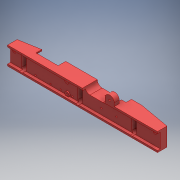
# Autodesk Inventor part: xtion_custom
Saved by Autodesk Inventor 2017 (Build 210142000, 142)
## iProperties
Created: 2016-11-20
Part Number: xtion_custom
Material: PC/ABS Plastic
Document SubType Name: Modeling
Designer: Alistair
Density: 0.357273 g/cm^3
Appearance: Smooth - Red
Author: Alistair
## iProperties of the stored document xtion_custom_3DPrint.ipt
Created: 2016-11-26
Part Number: xtion_custom_3DPrint
Material: Generic
Document SubType Name: Modeling
Designer: Alistair
Density: 1 g/cm^3
Appearance: Default
Author: Alistair
Autodesk Inventor part; units mm, degrees
ref_plane "YZ Plane" through (0, 0, 0) normal (1, 0, 0) x (0, 1, 0)
ref_plane "XZ Plane" through (0, 0, 0) normal (0, 1, 0) x (-1, 0, 0)
sketch "Sketch1" plane through (0, 0, 0) normal (0, 0, 1) x (1, 0, 0)
  line L0 (-10.5, 14) -> (-30.5, 14) projected
  line L1 (-30.5, 5.7) -> (-59, 5.7) construction
  line L2 (36.089, 8.08) -> (32.189, 8.08) projected
  line L3 (19.389, 8.08) -> (15.889, 8.08) projected
  line L4 (-10.5, 14) -> (14.0458, 14)
  line L5 (14.0458, 14) -> (14.0458, 8.08)
  line L6 (14.0458, 8.08) -> (15.889, 8.08)
  line L7 (19.389, 8.08) -> (19.389, 3.1279)
  line L8 (19.389, 3.1279) -> (32.189, 3.1279)
  line L9 (32.189, 3.1279) -> (32.189, 8.08)
  line L10 (36.089, 8.08) -> (37.2137, 8.08)
  line L11 (37.2137, 8.08) -> (37.2137, 14)
  line L12 (37.2137, 14) -> (48.426, 14)
  line L13 (48.426, 14) -> (82, 8.08)
  line L14 (82, 8.08) -> (82, -2.3)
  line L15 (82, -2.3) -> (-82, -2.3)
  line L16 (-82, -2.3) -> (-82, 8.08)
  line L17 (82, 0) -> (82, 29) projected
  line L18 (-82, 0) -> (-82, 29) projected
  line L19 (-82, 8.08) -> (-59, 12.1355)
  line L20 (-59, 5.7) -> (-59, 12.1355)
  line L21 (-34.7264, 5.7) -> (-34.7264, 14)
  line L22 (-34.7264, 14) -> (-30.5, 14)
  line L23 (-34.7264, 5.7) -> (-59, 5.7)
  line L24 (82, 8.08) -> (-65.0862, 8.08) construction
  point P0 (0, 0)
  dimension "d0" = 100
  dimension "d1" = 0
  dimension "d2" = 0
  dimension "d3" = 100
  dimension "d6" = 8
  constraints: 38 end point, 7 perpendicular, 6 point on line, 3 vertical, 2 collinear, 2 horizontal, 1 parallel
  measures "d0" angle of L13 L14
  measures "d1" distance between parallel lines of L14 L17
  measures "d2" distance between parallel lines of L16 L18
  measures "d3" angle of L19 L16
  measures "d6" distance between parallel lines of L15 L1
extrude "Extrusion1" add sketch "Sketch1" along normal mid plane 20
sketch "Sketch2" plane through (-82, -2.3, 10) normal (0, -1, 0) x (1, 0, 0)
  line L0 (164, -20) -> (164, 0) projected
  line L1 (0, 0) -> (164, 0) projected
  line L2 (0, -20) -> (0, 0) projected
  line L3 (164, -20) -> (0, -20) projected
  line L4 (0, -20) -> (0, 0) projected
  line L5 (0, -2) -> (164, -2)
  line L6 (164, -2) -> (164, -18)
  line L7 (164, -18) -> (0, -18)
  line L8 (0, -18) -> (0, -2)
  line L9 (82, -10) -> (90.9812, -10) construction
  point P0 (164, -10)
  dimension "d7" = 16
  constraints: 10 end point, 3 point on line, 2 horizontal, 2 parallel, 1 midpoint, 1 perpendicular
  measures "d7" distance between parallel lines of L5 L7
extrude "Extrusion2" cut sketch "Sketch2" against normal blind 3 contours L7 L2 L5 L0
sketch "Sketch3" plane through (-82, 0.7, 10) normal (0, -1, 0) x (1, 0, 0)
  circle A0 centre (5.4792, -3.8) radius 2
  line L0 (5.4792, -3.8) -> (159.4792, -3.8) construction
  circle A1 centre (159.4792, -3.8) radius 2
  line L1 (164, -2) -> (164, -18) projected
  line L2 (0, -2) -> (164, -2) projected
  line L3 (0, -18) -> (0, -2) projected
  line L4 (164, -18) -> (0, -18) projected
  point P0 (82, -10)
  dimension "d10" = 4
  dimension "d11" = 154
  dimension "d12" = 4
  dimension "d13" = 1.8
  constraints: 2 centre point, 2 end point, 1 coincident, 1 horizontal
  measures "d10" diameter of A0
  measures "d11" distance of L0.start L0.end
  measures "d12" diameter of A1
  measures "d13" distance between parallel lines of L0 L2
extrude "Extrusion3" add sketch "Sketch3" along normal blind 1.2 contours A0 L2 | L2 A0 | L2 A1 | A1 L2
sketch "Sketch4" plane through (-34.7264, 14, 10) normal (0, 1, 0) x (1, 0, 0)
  line L0 (0, 20) -> (0, 0) projected
  line L1 (48.7722, 0) -> (0, 0) projected
  line L2 (48.7722, 20) -> (48.7722, 0) projected
  line L3 (0, 20) -> (48.7722, 20) projected
  line L4 (27.8056, 3.9) -> (27.8056, 16.1) projected
  line L5 (30.6056, 16.1) -> (30.6056, 3.9) projected
  line L6 (29.2376, 3.9) -> (29.2376, 16.1) construction
  line L7 (31.7376, 3.9) -> (31.7376, 16.1)
  line L8 (26.7376, 16.1) -> (26.7376, 3.9)
  arc A0 (26.7376, 3.9) -> (31.7376, 3.9) centre (29.2376, 3.9) ccw
  arc A1 (31.7376, 16.1) -> (26.7376, 16.1) centre (29.2376, 16.1) ccw
  line L9 (86.9056, 15.85) -> (86.9056, 4.15) projected
  line L10 (89.9056, 4.15) -> (89.9056, 15.85) projected
  line L11 (-30.7944, 3.9) -> (-30.7944, 16.1) projected
  line L12 (-33.5944, 16.1) -> (-33.5944, 3.9) projected
  line L13 (88.3086, 4.15) -> (88.3086, 15.7466) construction
  line L14 (90.8086, 4.15) -> (90.8086, 15.7466)
  line L15 (85.8086, 15.7466) -> (85.8086, 4.15)
  arc A2 (85.8086, 4.15) -> (90.8086, 4.15) centre (88.3086, 4.15) ccw
  arc A3 (90.8086, 15.7466) -> (85.8086, 15.7466) centre (88.3086, 15.7466) ccw
  line L16 (-32.2263, 3.9) -> (-32.2263, 16.1) construction
  line L17 (-29.7263, 3.9) -> (-29.7263, 16.1)
  line L18 (-34.7263, 16.1) -> (-34.7263, 3.9)
  arc A4 (-34.7263, 3.9) -> (-29.7263, 3.9) centre (-32.2263, 3.9) ccw
  arc A5 (-29.7263, 16.1) -> (-34.7263, 16.1) centre (-32.2263, 16.1) ccw
  line L19 (41.7056, 2.5) -> (51.5556, 2.5) projected
  line L20 (66.9154, 0) -> (54.1154, 0) projected
  line L21 (54.1154, 0) -> (39.8429, 0) construction
  line L22 (48.7722, 0) -> (0, 0) projected
  line L23 (54.1154, -5.3087) -> (39.8429, -5.3087)
  line L24 (39.8429, 5.3087) -> (54.1154, 5.3087)
  arc A6 (54.1154, -5.3087) -> (54.1154, 5.3087) centre (54.1154, 0) ccw
  arc A7 (39.8429, 5.3087) -> (39.8429, -5.3087) centre (39.8429, 0) ccw
  point P0 (34.7264, 10)
  point P1 (29.2376, 10)
  point P2 (88.3086, 9.9483)
  point P3 (-32.2263, 10)
  point P4 (46.9792, 0)
  dimension "d16" = 5
  dimension "d19" = 5
  dimension "d20" = 5
  constraints: 32 end point, 16 point on circle, 16 tangent, 8 centre point, 5 parallel, 4 midpoint, 2 vertical, 1 point on line
  measures "d16" diameter of A1
  measures "d19" diameter of A3
  measures "d20" diameter of A5
extrude "Extrusion4" cut sketch "Sketch4" against normal through all contours A7 L24 L2 L1 | L1 L2 L24 A6 L23 A7 | A0 L8 A1 L7 | A2 L15 A3 L14 | A4 L18 A5 L17
sketch "Sketch5" plane through (-34.7264, 14, -10) normal (0, 1, 0) x (1, 0, 0)
  line L0 (71.9401, 0) -> (71.9401, -20) projected
  line L1 (83.1524, -20) -> (71.9401, -20) projected
  line L2 (83.1524, 0) -> (83.1524, -20) projected
  line L3 (71.9401, 0) -> (83.1524, 0) projected
  line L4 (39.8429, -14.6913) -> (48.7722, -14.6913) projected
  line L5 (48.7722, 0) -> (48.7722, -14.6913) projected
  line L6 (0, 0) -> (48.7722, 0) projected
  line L7 (0, 0) -> (0, -20) projected
  line L8 (34.5342, -20) -> (0, -20) projected
  arc A0 (39.8429, -14.6913) -> (34.5342, -20) centre (39.8429, -20) ccw projected
  arc A1 (31.7376, -3.9) -> (26.7376, -3.9) centre (29.2376, -3.9) ccw projected
  line L9 (31.7376, -3.9) -> (31.7376, -16.1) projected
  arc A2 (26.7376, -16.1) -> (31.7376, -16.1) centre (29.2376, -16.1) ccw projected
  line L10 (26.7376, -16.1) -> (26.7376, -3.9) projected
  line L11 (71.9401, 0) -> (48.7722, 0)
  line L12 (48.7722, 0) -> (48.7722, -3.6)
  line L13 (48.7722, -3.6) -> (71.9401, -3.6)
  line L14 (71.9401, -3.6) -> (71.9401, 0)
  point P0 (34.7264, -10)
  dimension "d21" = 3.6
  constraints: 8 end point, 2 parallel, 1 horizontal, 1 perpendicular, 1 point on line
  measures "d21" distance between parallel lines of L11 L13
extrude "Extrusion5" add sketch "Sketch5" against normal up to surface (10.8721 mm away) contours L0 L13 L5 L11
fillet "Fillet1" radius 3 2 edges at (14.0458, 11.04, -6.4) (37.2137, 11.04, -6.4)
sketch "Sketch6" plane through (-82, 0.7, 10) normal (0, -1, 0) x (1, 0, 0)
  circle A0 centre (62.9792, -3.8) radius 0.95 projected
  circle A1 centre (62.9792, -16.2) radius 0.95 projected
  circle A2 centre (62.9792, -3.8) radius 2.5
  circle A3 centre (62.9792, -16.2) radius 2.5
  point P0 (82, -10)
  dimension "d25" = 5
  dimension "d26" = 5
  constraints: 2 centre point, 2 coincident
  measures "d25" diameter of A2
  measures "d26" diameter of A3
ref_plane "Work Plane1" through (-78.5208, -0.5, -8) normal (0, 1, 0) x (0, 0, 1)
extrude "Extrusion6" add sketch "Sketch6" along normal up to surface (1.2 mm away) contours A0 | A1 | A2 | A3
sketch "Sketch7" plane through (82, -2.3, 8) normal (0, -1, 0) x (1, 0, 0)
  arc A0 (-27.1421, 0) -> (-29.6935, 0) centre (-28.4178, -2.15) ccw projected
  line L0 (-27.1421, 0) -> (0, 0) projected
  line L1 (0, 0) -> (0, 2) projected
  line L2 (-57.3023, 2) -> (0, 2) projected
  arc A1 (-57.6935, 0) -> (-57.3023, 2) centre (-62.611, 2) ccw projected
  line L3 (-57.6935, 0) -> (-29.6935, 0) projected
  line L4 (-57.3023, 2) -> (0, 2) projected
  line L5 (-52.3023, 2) -> (-52.3023, 5.5935) construction
  line L6 (-57.3023, 2) -> (-57.3023, 5.5935)
  line L7 (-47.3023, 5.5935) -> (-47.3023, 2)
  arc A2 (-57.3023, 2) -> (-47.3023, 2) centre (-52.3023, 2) ccw
  arc A3 (-47.3023, 5.5935) -> (-57.3023, 5.5935) centre (-52.3023, 5.5935) ccw
  line L8 (-57.3023, 2) -> (-47.3023, 2)
  line L9 (-44.7863, 2) -> (-49.811, 2) projected
  arc A4 (-57.6935, 0) -> (-57.3023, 2) centre (-62.611, 2) ccw projected
  point P0 (-82, -8)
  point P1 (-52.3023, 3.7968)
  dimension "d31" = 10
  constraints: 10 end point, 5 tangent, 4 point on circle, 2 centre point, 1 collinear, 1 midpoint, 1 parallel, 1 perpendicular, 1 point on line
  measures "d31" distance between parallel lines of L7 L6
extrude "Extrusion7" add sketch "Sketch7" against normal up to surface (5.4279 mm away) contours L2 L6 A3 L7
sketch "Sketch8" plane through (-34.7264, 14, -10) normal (0, 1, 0) x (1, 0, 0)
  circle A0 centre (68.8654, -8.6) radius 1
  circle A1 centre (52.3654, -8.6) radius 1
  circle A2 centre (20.7264, -3.75) radius 1 projected
  circle A3 centre (20.7264, -16.25) radius 1 projected
  circle A4 centre (7.7264, -16.25) radius 1 projected
  circle A5 centre (7.7264, -3.75) radius 1 projected
  circle A6 centre (-3.2253, -3.7134) radius 1 projected
  circle A7 centre (-3.2737, -16.3134) radius 1 projected
  circle A8 centre (-19.7736, -16.25) radius 1 projected
  circle A9 centre (-19.7252, -3.6501) radius 1 projected
  line L0 (39.8429, -14.6913) -> (48.7722, -14.6913) projected
  line L1 (48.7722, -6.6) -> (48.7722, -14.6913) projected
  arc A10 (51.7722, -3.6) -> (48.7722, -6.6) centre (51.7722, -6.6) ccw projected
  line L2 (51.7722, -3.6) -> (68.9401, -3.6) projected
  arc A11 (71.9401, -6.6) -> (68.9401, -3.6) centre (68.9401, -6.6) ccw projected
  line L3 (71.9401, -6.6) -> (71.9401, -20) projected
  line L4 (83.1524, -20) -> (71.9401, -20) projected
  line L5 (83.1524, 0) -> (83.1524, -20) projected
  line L6 (0, 0) -> (83.1524, 0) projected
  line L7 (0, 0) -> (0, -20) projected
  line L8 (34.5342, -20) -> (0, -20) projected
  arc A12 (39.8429, -14.6913) -> (34.5342, -20) centre (39.8429, -20) ccw projected
  arc A13 (31.7376, -3.9) -> (26.7376, -3.9) centre (29.2376, -3.9) ccw projected
  line L9 (31.7376, -3.9) -> (31.7376, -16.1) projected
  arc A14 (26.7376, -16.1) -> (31.7376, -16.1) centre (29.2376, -16.1) ccw projected
  line L10 (26.7376, -16.1) -> (26.7376, -3.9) projected
  line L11 (-24.2736, 0) -> (-24.2736, -20) projected
  line L12 (0, -20) -> (-24.2736, -20) projected
  line L13 (0, 0) -> (0, -20) projected
  line L14 (-24.2736, 0) -> (0, 0) projected
  line L15 (68.8654, -8.6) -> (52.3654, -8.6) construction
  point P0 (34.7264, -10)
  dimension "d67" = 16.5
  dimension "d68" = 5
  constraints: 10 coincident, 2 centre point, 2 end point, 1 horizontal
  measures "d67" distance of L15.start L15.end
  measures "d68" distance between parallel lines of L2 L15
hole "Hole1" at (34.139, 14, -1.4) at (17.639, 14, -1.4) at (-14, 14, 6.25) at (-14, 14, -6.25) at (-27, 14, -6.25) at (-27, 14, 6.25) at (-38.0001, 14, 6.3134) at (-37.9517, 14, -6.2866) at (-54.4516, 14, -6.3499) at (-54.5, 14, 6.25) direction (0, -1, 0) diameter 1.4 end through all
hole "Hole2" at (29.6977, -2.3, 13.5935) direction (0, 1, 0) diameter 1.8 end through all
sketch "Sketch9" plane through (14.0458, 8.08, 4.6913) normal (0, 1, 0) x (1, 0, 0)
  line L0 (5.0432, 2.5913) -> (1.0432, 2.5913) projected
  line L1 (5.0432, 6.7913) -> (1.0432, 6.7913) projected
  line L2 (7.0432, 1.3913) -> (14.8432, 1.3913) projected
  line L3 (14.8432, 1.3913) -> (14.8432, 7.9913) projected
  line L4 (14.8432, 7.9913) -> (7.0432, 7.9913) projected
  line L5 (7.0432, 7.9913) -> (7.0432, 1.3913) projected
  circle A0 centre (3.5932, 4.6913) radius 1 projected
  arc A1 (1.0486, 1.3413) -> (3.1432, -0.6087) centre (3.1432, 1.4913) ccw projected
  line L6 (1.0486, 1.3413) -> (5.0432, 1.3413) projected
  line L7 (5.0432, 1.3413) -> (5.0432, 2.5913) projected
  line L8 (5.0432, 2.5913) -> (1.0432, 2.5913) projected
  line L9 (1.0432, 2.5913) -> (1.0432, 6.7913) projected
  line L10 (1.0432, 6.7913) -> (5.0432, 6.7913) projected
  line L11 (5.0432, 6.7913) -> (5.0432, 8.0413) projected
  line L12 (5.0432, 8.0413) -> (1.0486, 8.0413) projected
  arc A2 (3.1432, 9.9913) -> (1.0486, 8.0413) centre (3.1432, 7.8913) ccw projected
  line L13 (3.1432, 9.9913) -> (16.9432, 9.9913) projected
  line L14 (16.9432, 9.9913) -> (16.9432, -0.6087) projected
  line L15 (16.9432, -0.6087) -> (3.1432, -0.6087) projected
  line L16 (1.0486, 3.375) -> (6.44, 3.375) construction
  line L17 (5.3432, 11.0913) -> (5.3432, 0) projected
  line L18 (1.0486, 2.575) -> (6.44, 2.575)
  line L19 (6.44, 4.175) -> (1.0486, 4.175)
  arc A3 (1.0486, 4.175) -> (1.0486, 2.575) centre (1.0486, 3.375) ccw
  arc A4 (6.44, 2.575) -> (6.44, 4.175) centre (6.44, 3.375) ccw
  line L20 (1.0486, 8.825) -> (6.44, 8.825) construction
  line L21 (1.0486, 8.025) -> (6.44, 8.025)
  line L22 (6.44, 9.625) -> (1.0486, 9.625)
  arc A5 (1.0486, 9.625) -> (1.0486, 8.025) centre (1.0486, 8.825) ccw
  arc A6 (6.44, 8.025) -> (6.44, 9.625) centre (6.44, 8.825) ccw
  point P0 (-14.0458, 4.6913)
  point P1 (3.7443, 3.375)
  point P2 (3.7443, 8.825)
  dimension "d48" = 1.6
  dimension "d49" = 1.6
  constraints: 16 end point, 8 point on circle, 8 tangent, 4 centre point, 3 parallel, 2 midpoint, 1 perpendicular
  measures "d48" diameter of A4
  measures "d49" diameter of A6
extrude "Extrusion8" cut sketch "Sketch9" against normal blind 2 contours L7 L18 A3 L9 L0 | L0 L9 A3 L19 A0 L17 L18 L7 | L17 L19 A4 L5 L18 | L19 A0 | L21 L11 L12 A2 L22 L17 | L17 L22 A6 L21 | L5 A4 | L21 A5 L22 A2 L12 L11 picked at (3.4812, 4.0332)
sketch "Sketch10" plane through (-34.7264, 14, -10) normal (0, 1, 0) x (1, 0, 0)
  line L0 (89.9056, -4.15) -> (86.9056, -4.15) projected
  line L1 (86.9056, -4.15) -> (86.9056, -15.85) projected
  line L2 (86.9056, -15.85) -> (89.9056, -15.85) projected
  line L3 (89.9056, -15.85) -> (89.9056, -4.15) projected
  line L4 (86.9056, -13.6) -> (65.3423, -13.6)
  line L5 (65.3423, -13.6) -> (65.3423, -3.6)
  line L6 (65.3423, -3.6) -> (86.9056, -3.6)
  line L7 (86.9056, -3.6) -> (86.9056, -15.85)
  line L8 (86.9056, -13.6) -> (86.9056, -3.6)
  circle A0 centre (68.8654, -8.6) radius 0.7 projected
  line L9 (68.8654, -8.6) -> (71.0081, -8.6) construction
  point P0 (34.7264, -10)
  point P1 (65.3423, -8.6)
  dimension "d54" = 10
  constraints: 12 end point, 2 horizontal, 2 parallel, 1 midpoint, 1 perpendicular, 1 point on line, 1 vertical
  measures "d54" distance between parallel lines of L6 L4
extrude "Extrusion9" cut sketch "Sketch10" against normal up to surface (5.92 mm away) contours L1 L4 L5 L6 L7 | A0
sketch "Sketch11" plane through (-34.7264, 14, -10) normal (0, 1, 0) x (1, 0, 0)
  arc A0 (-29.7263, -3.9) -> (-34.7263, -3.9) centre (-32.2263, -3.9) ccw projected
  line L0 (-29.7263, -3.9) -> (-29.7263, -16.1) projected
  arc A1 (-34.7263, -16.1) -> (-29.7263, -16.1) centre (-32.2263, -16.1) ccw projected
  line L1 (-34.7263, -16.1) -> (-34.7263, -3.9) projected
  line L2 (-47.2736, 0) -> (-47.2736, -20) projected
  line L3 (-24.2736, -20) -> (-47.2736, -20) projected
  line L4 (-24.2736, 0) -> (-24.2736, -20) projected
  line L5 (-47.2736, 0) -> (-24.2736, 0) projected
  arc A2 (-33.8511, -18) -> (-30.6015, -18) centre (-32.2263, -16.1) ccw projected
  line L6 (-32.2263, -18.6) -> (-22.9234, -18.6)
  line L7 (-30.6015, -18) -> (27.6128, -18) projected
  line L8 (-22.9234, -18.6) -> (-22.9234, -1.4)
  line L9 (-22.9234, -1.4) -> (-32.2263, -1.4)
  arc A3 (-30.6015, -2) -> (-33.8511, -2) centre (-32.2263, -3.9) ccw projected
  point P0 (34.7264, -10)
  constraints: 6 end point, 4 point on circle, 1 parallel, 1 perpendicular
extrude "Extrusion10" cut sketch "Sketch11" against normal up to surface (8.3 mm away) contours L0 A1 L1 A0 | A0 L9 L4 L7 A1 L0 | L7 L4 L6 A1 | L9 L8 L7 L4 | L7 L8 L6 L4
fillet "Fillet2" radius 4 1 edges at (51.0822, 10.8058, 3.6)
fillet "Fillet3" radius 4 3 edges at (51.104, 8.08, -6.0762) (51.1054, 8.08, 6.1897) (51.0822, 8.08, 0.0517)
fillet "Fillet4" radius 2 3 edges at (-65.1849, 5.7, -7.8678) (-65.1849, 5.7, 7.8678) (-64.4527, 5.7, 0)
sketch "Sketch12" plane through (-82, -0.5, 10) normal (0, -1, 0) x (1, 0, 0)
  line L0 (4.6074, -2) -> (6.351, -2) projected
  arc A0 (4.6074, -2) -> (6.351, -2) centre (5.4792, -3.8) ccw projected
  line L1 (61.2443, -2) -> (64.7142, -2) projected
  arc A1 (61.2443, -2) -> (64.7142, -2) centre (62.9792, -3.8) ccw projected
  line L2 (64.7142, -18) -> (61.2443, -18) projected
  arc A2 (64.7142, -18) -> (61.2443, -18) centre (62.9792, -16.2) ccw projected
  line L3 (158.6074, -2) -> (160.351, -2) projected
  arc A3 (158.6074, -2) -> (160.351, -2) centre (159.4792, -3.8) ccw projected
  point P0 (82, -10)
  constraints: 4 coincident
hole "Hole3" at (-76.5208, -0.5, 6.2) at (-19.0208, -0.5, 6.2) at (-19.0208, -0.5, -6.2) at (77.4792, -0.5, 6.2) direction (0, 1, 0) diameter 1.4 depth 8 tip angle 118
equation "\"d3\" = d0"
equation "\"d10\" = d12"
body "Solid1"
